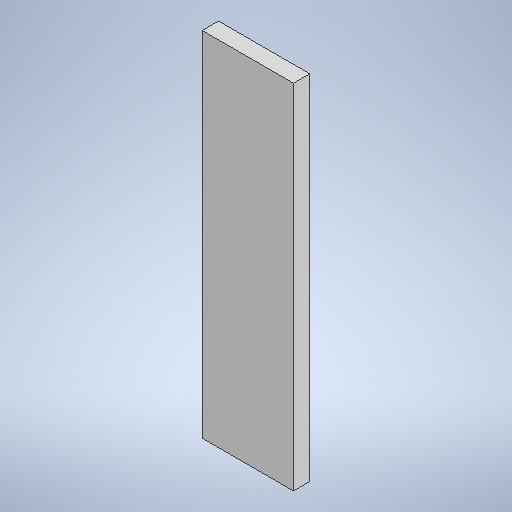
# Autodesk Inventor part: carcasa_piezaLateral_frontal
Saved by Autodesk Inventor 2025.3 (Build 293356030, 356C)
## iProperties
Created: 2025-09-08
Part Number: carcasa_piezaLateral_frontal
Material: Generic
Document SubType Name: Modeling
Designer: brene
Density: 1 g/cm^3
Appearance: Default
Author: brene
Autodesk Inventor part; units mm, degrees
ref_plane "YZ Plane" through (0, 0, 0) normal (1, 0, 0) x (0, 1, 0)
ref_plane "XZ Plane" through (0, 0, 0) normal (0, 1, 0) x (-1, 0, 0)
ref_plane "XY Plane" through (0, 0, 0) normal (0, 0, 1) x (1, 0, 0)
sketch "Sketch1" plane through (0, 0, 0) normal (0, 0, 1) x (1, 0, 0)
  line L0 (0, 0) -> (16.8, 0)
  line L1 (16.8, 0) -> (16.8, 65)
  line L2 (16.8, 65) -> (0, 65)
  line L3 (0, 65) -> (0, 0)
  dimension "d0" = 16.8
  dimension "d1" = 65
  dimension "d2" = 16.8
  constraints: 8 end point, 2 perpendicular, 1 horizontal
  measures "d0" distance of L0.start L0.end
  measures "d1" distance of L0.end L1.end
  measures "d2" distance of L1.end L2.end
extrude "Extrusion1" add sketch "Sketch1" along normal blind 3
body "Solid1"
